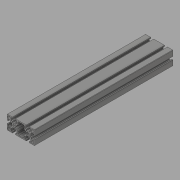
# Autodesk Inventor part: SW200
Saved by Autodesk Inventor 2021.3 (Build 253353000, 353)
## iProperties
Created: 2019-12-14
Part Number: SW200
Material: アルミニウム 6061
Document SubType Name: Modeling
Designer: gisen
Density: 2.7 g/cm^3
Appearance: アルミニウム - フラット
Sending System: Autodesk Inventor 2014
MC: AMD64
MC_MODEL: Intel64 Family 6 Model 94 Stepping 3, GenuineIntel
OS: Windows_NT
OS_RELEASE: 6.1
FRU: Autodesk
FORMAT: text
GUISE: transmit
KEY: AFS-2040-4
FILE: C:\Users\AMS43\Documents\Inventor\AMS\Inventor作成モデル\parasolidモデル\AFS-2040-4.x_t
DATE: Tue, 23 Aug 2016 16:58:34 GMT
Author: gisen
Autodesk Inventor part; units mm, degrees
ref_plane "YZ Plane" through (0, 0, 0) normal (1, 0, 0) x (0, 1, 0)
ref_plane "XZ Plane" through (0, 0, 0) normal (0, 1, 0) x (-1, 0, 0)
ref_plane "XY Plane" through (0, 0, 0) normal (0, 0, 1) x (1, 0, 0)
sketch "スケッチ1" plane through (-7.85, -10, 0) normal (0, 0, 1) x (1, 0, 0)
  line L0 (-6.3, 14.8) -> (-6.3, 18.5) projected
  line L1 (0, 13) -> (-4.3, 13) projected
  line L2 (-4.3, 13) -> (-4.3, 14.8) projected
  line L3 (-4.3, 14.8) -> (-6.3, 14.8) projected
  line L4 (-6.3, 14.8) -> (-6.3, 18.5) projected
  line L5 (-6.3, 18.5) -> (-4.3, 18.5) projected
  line L6 (-4.3, 18.5) -> (-4.3, 20) projected
  line L7 (-4.3, 20) -> (-11.65, 20) projected
  arc A0 (-11.65, 20) -> (-12.15, 19.5) centre (-11.65, 19.5) ccw projected
  line L8 (-12.15, 19.5) -> (-12.15, 12.15) projected
  line L9 (-12.15, 12.15) -> (-10.65, 12.15) projected
  line L10 (-10.65, 12.15) -> (-10.65, 14.15) projected
  line L11 (-10.65, 14.15) -> (-6.95, 14.15) projected
  line L12 (-6.95, 14.15) -> (-6.95, 12.15) projected
  line L13 (-6.95, 12.15) -> (-5.15, 12.15) projected
  line L14 (-5.15, 12.15) -> (-5.15, 7.85) projected
  line L15 (-5.15, 7.85) -> (-6.95, 7.85) projected
  line L16 (-6.95, 7.85) -> (-6.95, 5.85) projected
  line L17 (-6.95, 5.85) -> (-10.65, 5.85) projected
  line L18 (-10.65, 5.85) -> (-10.65, 7.85) projected
  line L19 (-10.65, 7.85) -> (-12.15, 7.85) projected
  line L20 (-12.15, 7.85) -> (-12.15, 0.5) projected
  arc A1 (-12.15, 0.5) -> (-11.65, 0) centre (-11.65, 0.5) ccw projected
  line L21 (-11.65, 0) -> (-4.3, 0) projected
  line L22 (-4.3, 0) -> (-4.3, 1.5) projected
  line L23 (-4.3, 1.5) -> (-6.3, 1.5) projected
  line L24 (-6.3, 1.5) -> (-6.3, 5.2) projected
  line L25 (-6.3, 5.2) -> (-4.3, 5.2) projected
  line L26 (-4.3, 5.2) -> (-4.3, 7) projected
  line L27 (-4.3, 7) -> (0, 7) projected
  line L28 (0, 7) -> (0, 5.2) projected
  line L29 (0, 5.2) -> (2, 5.2) projected
  line L30 (2, 5.2) -> (2, 1.5) projected
  line L31 (2, 1.5) -> (0, 1.5) projected
  line L32 (0, 1.5) -> (0, 0) projected
  line L33 (0, 0) -> (15.7, 0) projected
  line L34 (15.7, 0) -> (15.7, 1.5) projected
  line L35 (15.7, 1.5) -> (13.7, 1.5) projected
  line L36 (13.7, 1.5) -> (13.7, 5.2) projected
  line L37 (13.7, 5.2) -> (15.7, 5.2) projected
  line L38 (15.7, 5.2) -> (15.7, 7) projected
  line L39 (15.7, 7) -> (20, 7) projected
  line L40 (20, 7) -> (20, 5.2) projected
  line L41 (20, 5.2) -> (22, 5.2) projected
  line L42 (22, 5.2) -> (22, 1.5) projected
  line L43 (22, 1.5) -> (20, 1.5) projected
  line L44 (20, 1.5) -> (20, 0) projected
  line L45 (20, 0) -> (27.35, 0) projected
  arc A2 (27.35, 0) -> (27.85, 0.5) centre (27.35, 0.5) ccw projected
  line L46 (27.85, 0.5) -> (27.85, 7.85) projected
  line L47 (27.85, 7.85) -> (26.35, 7.85) projected
  line L48 (26.35, 7.85) -> (26.35, 5.85) projected
  line L49 (26.35, 5.85) -> (22.65, 5.85) projected
  line L50 (22.65, 5.85) -> (22.65, 7.85) projected
  line L51 (22.65, 7.85) -> (20.85, 7.85) projected
  line L52 (20.85, 7.85) -> (20.85, 12.15) projected
  line L53 (20.85, 12.15) -> (22.65, 12.15) projected
  line L54 (22.65, 12.15) -> (22.65, 14.15) projected
  line L55 (22.65, 14.15) -> (26.35, 14.15) projected
  line L56 (26.35, 14.15) -> (26.35, 12.15) projected
  line L57 (26.35, 12.15) -> (27.85, 12.15) projected
  line L58 (27.85, 12.15) -> (27.85, 19.5) projected
  arc A3 (27.85, 19.5) -> (27.35, 20) centre (27.35, 19.5) ccw projected
  line L59 (27.35, 20) -> (20, 20) projected
  line L60 (20, 20) -> (20, 18.5) projected
  line L61 (20, 18.5) -> (22, 18.5) projected
  line L62 (22, 18.5) -> (22, 14.8) projected
  line L63 (22, 14.8) -> (20, 14.8) projected
  line L64 (20, 14.8) -> (20, 13) projected
  line L65 (20, 13) -> (15.7, 13) projected
  line L66 (15.7, 13) -> (15.7, 14.8) projected
  line L67 (15.7, 14.8) -> (13.7, 14.8) projected
  line L68 (13.7, 14.8) -> (13.7, 18.5) projected
  line L69 (13.7, 18.5) -> (15.7, 18.5) projected
  line L70 (15.7, 18.5) -> (15.7, 20) projected
  line L71 (15.7, 20) -> (0, 20) projected
  line L72 (0, 20) -> (0, 18.5) projected
  line L73 (0, 18.5) -> (2, 18.5) projected
  line L74 (2, 18.5) -> (2, 14.8) projected
  line L75 (2, 14.8) -> (0, 14.8) projected
  line L76 (0, 14.8) -> (0, 13) projected
  line L77 (12.35, 17) -> (12.35, 14.9075) projected
  arc A4 (12.35, 14.9075) -> (13.85, 12.3094) centre (15.35, 14.9075) ccw projected
  line L78 (13.85, 12.3094) -> (16.0391, 11.0455) projected
  arc A5 (16.0391, 11.0455) -> (16.6521, 11.1347) centre (16.2891, 11.4785) ccw projected
  arc A6 (16.6521, 8.8653) -> (16.6521, 11.1347) centre (17.85, 10) ccw projected
  arc A7 (16.6521, 8.8653) -> (16.0391, 8.9545) centre (16.2891, 8.5215) ccw projected
  line L79 (16.0391, 8.9545) -> (13.85, 7.6906) projected
  arc A8 (13.85, 7.6906) -> (12.35, 5.0925) centre (15.35, 5.0925) ccw projected
  line L80 (12.35, 5.0925) -> (12.35, 3) projected
  arc A9 (10.85, 1.5) -> (12.35, 3) centre (10.85, 3) ccw projected
  line L81 (10.85, 1.5) -> (4.85, 1.5) projected
  arc A10 (3.35, 3) -> (4.85, 1.5) centre (4.85, 3) ccw projected
  line L82 (3.35, 3) -> (3.35, 5.0925) projected
  arc A11 (3.35, 5.0925) -> (1.85, 7.6906) centre (0.35, 5.0925) ccw projected
  line L83 (1.85, 7.6906) -> (-0.3391, 8.9545) projected
  arc A12 (-0.3391, 8.9545) -> (-0.9521, 8.8653) centre (-0.5891, 8.5215) ccw projected
  arc A13 (-0.9521, 11.1347) -> (-0.9521, 8.8653) centre (-2.15, 10) ccw projected
  arc A14 (-0.9521, 11.1347) -> (-0.3391, 11.0455) centre (-0.5891, 11.4785) ccw projected
  line L84 (-0.3391, 11.0455) -> (1.85, 12.3094) projected
  arc A15 (1.85, 12.3094) -> (3.35, 14.9075) centre (0.35, 14.9075) ccw projected
  line L85 (3.35, 14.9075) -> (3.35, 17) projected
  arc A16 (4.85, 18.5) -> (3.35, 17) centre (4.85, 17) ccw projected
  line L86 (4.85, 18.5) -> (10.85, 18.5) projected
  arc A17 (12.35, 17) -> (10.85, 18.5) centre (10.85, 17) ccw projected
  circle A18 centre (24.85, 3) radius 2 projected
  circle A19 centre (-9.15, 3) radius 2 projected
  circle A20 centre (-9.15, 17) radius 2 projected
  circle A21 centre (24.85, 17) radius 2 projected
  point P0 (7.85, 10)
extrude "押し出し1" add sketch "スケッチ1" along normal blind 200
equation "\"d0\" = L"
equation "\"L\" = 200"
